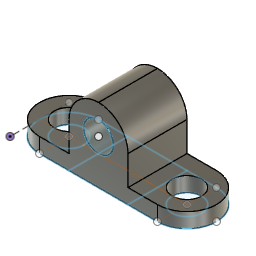
A4 (Autodesk Fusion 360 design; units mm, degrees)
Autodesk Fusion 360 part; units mm, degrees
sketch "Base" plane through (0, 0, 0) normal (0, 0, 1) x (1, 0, 0)
  line L0 (0, 0) -> (0, 20) construction
  line L1 (0, 20) -> (0, 40) construction
  line L2 (0, 20) -> (120, 20) construction
  line L3 (20, 20) -> (20, 0) construction
  line L4 (20, 20) -> (20, 40) construction
  line L5 (100, 20) -> (100, 40) construction
  line L6 (100, 20) -> (100, 0) construction
  line L7 (20, 0) -> (100, 0)
  arc A0 (100, 0) -> (100, 40) centre (100, 20) ccw
  line L8 (100, 40) -> (20, 40)
  arc A1 (20, 40) -> (20, 0) centre (20, 20) ccw
  line L9 (20, 20) -> (100, 20) construction
  circle A2 centre (20, 20) radius 10
  circle A3 centre (100, 20) radius 10
  line L10 (40, 40) -> (40, 0)
  line L11 (80, 40) -> (80, 0)
  constraint coincident L0.start origin
  constraint vertical L0
  constraint parallel L0 L1
  constraint perpendicular L0 L2
  constraint coincident L2 L3.start
  constraint coincident L2 L5.start
  constraint perpendicular L2 L5
  constraint perpendicular L2 L6
  constraint tangent L7 A0
  constraint tangent A0 L8
  constraint parallel L7 L8
  constraint tangent L8 A1
  constraint tangent L7 A1
  constraint coincident L5.start L6.start
  constraint perpendicular L5 L9
  constraint coincident L3.start L4.start
  constraint concentric A1 A2
  constraint concentric A0 A3
  constraint coincident L8 L10.start
  constraint coincident L7 L10.end
  constraint perpendicular L7 L10
  constraint coincident L8 L11.start
  constraint coincident L7 L11.end
  constraint perpendicular L7 L11
extrude "Extrude1" add sketch "Base" along normal blind 10
extrude "Extrude2" add sketch "Base" along normal blind 50 contours L7 L8 L10 L11
fillet "Fillet1" radius 20 2 edges at (80, 20, 50) (40, 20, 50)
sketch "Circle" plane through (0, 0, 0) normal (0, 1, 0) x (1, 0, 0)
  circle A0 centre (60, -30) radius 10
extrude "Extrude3" cut sketch "Circle" along normal blind 40
named bodies: "MainBodyA4"
